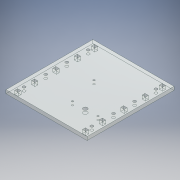
# Autodesk Inventor part: Plano 2
Saved by Autodesk Inventor 2018 (Build 220112000, 112)
## iProperties
Created: 2017-08-31
Part Number: Plano 2
Material: Vidrio
Document SubType Name: Modeling
Designer: Alumno
Density: 2.18 g/cm^3
Appearance: Claro
Author: Alumno
Autodesk Inventor part; units mm, degrees
ref_plane "YZ Plane" through (0, 0, 0) normal (1, 0, 0) x (0, 1, 0)
ref_plane "XZ Plane" through (0, 0, 0) normal (0, 1, 0) x (-1, 0, 0)
ref_plane "XY Plane" through (0, 0, 0) normal (0, 0, 1) x (1, 0, 0)
sketch "Boceto1" plane through (0, 0, 0) normal (0, 0, 1) x (1, 0, 0)
  line L0 (70, -75) -> (-70, -75)
  line L1 (-70, -75) -> (-70, 75)
  line L2 (-70, 75) -> (70, 75)
  line L3 (70, 75) -> (70, -75)
  line L4 (70, -75) -> (-70, 75) construction
  line L5 (-70, -75) -> (70, 75) construction
  point P0 (0, 0)
  dimension "d0" = 140
  dimension "d1" = 150
  constraints: 12 end point, 2 midpoint, 2 parallel, 1 horizontal, 1 perpendicular
  measures "d0" distance of L1.end L2.end
  measures "d1" distance of L0.end L1.end
extrude "Extrusión1" add sketch "Boceto1" along normal blind 6
sketch "Boceto2" plane through (0, 0, 6) normal (0, 0, 1) x (1, 0, 0)
  line L0 (-70, -75) -> (70, -75) projected
  line L1 (70, -75) -> (70, 75) projected
  line L2 (70, 75) -> (-70, 75) projected
  line L3 (-70, 75) -> (-70, -75) projected
  line L4 (70, 75) -> (70, 68.9297)
  line L5 (70, 63.9297) -> (70, 57)
  line L6 (70, 53.65) -> (70, 39.3833)
  line L7 (70, 34.3833) -> (70, 20.1167)
  line L8 (70, 16.7667) -> (70, 2.5)
  line L9 (70, -2.5) -> (70, -16.7667)
  line L10 (70, -20.1167) -> (70, -34.3833)
  line L11 (70, 75) -> (70, 68.9297)
  line L12 (61.5, 68.9297) -> (61.5, 63.9297)
  line L13 (70, 63.9297) -> (70, 57)
  line L14 (70, 53.65) -> (70, 39.3833)
  line L15 (70, 34.3833) -> (70, 20.1167)
  line L16 (70, 16.7667) -> (70, 2.5)
  line L17 (61.5, 2.5) -> (61.5, -2.5)
  line L18 (70, -2.5) -> (70, -16.7667)
  line L19 (70, -20.1167) -> (70, -34.3833)
  line L20 (61.5, -34.3833) -> (61.5, -39.3833)
  line L21 (61.5, -63.5) -> (61.5, -68.5)
  line L22 (61.5, 68.9297) -> (55.5, 68.9297)
  line L23 (55.5, 68.9297) -> (55.5, 63.9297)
  line L24 (55.5, 63.9297) -> (61.5, 63.9297)
  line L25 (61.5, 63.9297) -> (61.5, 68.9297)
  line L26 (61.5, 34.3833) -> (55.5, 34.3833)
  line L27 (55.5, 34.3833) -> (55.5, 39.3833)
  line L28 (55.5, 39.3833) -> (61.5, 39.3833)
  line L29 (61.5, 39.3833) -> (61.5, 34.3833)
  line L30 (55.5, 2.5) -> (61.5, 2.5)
  line L31 (61.5, 2.5) -> (61.5, -2.5)
  line L32 (61.5, -2.5) -> (55.5, -2.5)
  line L33 (55.5, -2.5) -> (55.5, 2.5)
  line L34 (55.5, -34.3833) -> (61.5, -34.3833)
  line L35 (61.5, -34.3833) -> (61.5, -39.3833)
  line L36 (61.5, -39.3833) -> (55.5, -39.3833)
  line L37 (55.5, -39.3833) -> (55.5, -34.3833)
  line L38 (55.5, -68.5) -> (61.5, -68.5)
  line L39 (61.5, -68.5) -> (61.5, -63.5)
  line L40 (61.5, -63.5) -> (55.5, -63.5)
  line L41 (55.5, -63.5) -> (55.5, -68.5)
  dimension "d7" = 5
  dimension "d8" = 6
  dimension "d9" = 5
  dimension "d12" = 6
  dimension "d16" = 6
  dimension "d35" = 8.5
  dimension "d36" = 6
  dimension "d37" = 8.5
  dimension "d40" = 8.5
  dimension "d45" = 8.5
  dimension "d46" = 8.5
  dimension "d47" = 6
  dimension "d48" = 5
  dimension "d49" = 5
  dimension "d50" = 5
  constraints: 76 end point, 10 parallel, 5 horizontal, 5 perpendicular, 2 coincident
  measures "d7" distance of L23.end L22.end
  measures "d8" distance of L27.end L28.end
  measures "d9" distance of L26.end L27.end
  measures "d12" distance of L17.end L32.end
  measures "d16" distance of L20.end L36.end
  measures "d35" distance between parallel lines of L1 L12
  measures "d36" distance of L12.start L22.end
  measures "d37" distance between parallel lines of L1 L29
  measures "d40" distance between parallel lines of L1 L17
  measures "d45" distance between parallel lines of L20 L1
  measures "d46" distance between parallel lines of L1 L21
  measures "d47" distance of L21.start L40.end
  measures "d48" distance of L40.end L38.start
  measures "d49" distance of L20.start L20.end
  measures "d50" distance of L32.end L30.start
extrude "Extrusión2" cut sketch "Boceto2" against normal blind 6 contours L12 L24 L23 L22 | L17 L32 L33 L30 | L20 L36 L37 L34 | L21 L38 L41 L40 | L26 L27 L28 L29
mirror "Simetría1" about plane through (0, 0, 0) normal (1, 0, 0) of "Extrusión2"
sketch "Boceto4" plane through (0, 0, 6) normal (0, 0, 1) x (1, 0, 0)
  line L0 (70, 75) -> (70, 68.9297)
  line L1 (70, 68.9297) -> (65, 68.9297)
  line L2 (65, 68.9297) -> (65, 63.9297)
  line L3 (65, 63.9297) -> (70, 63.9297)
  line L4 (70, 63.9297) -> (70, 57)
  line L5 (70, 53.65) -> (70, 39.3833)
  line L6 (70, 39.3833) -> (65, 39.3833)
  line L7 (65, 39.3833) -> (65, 34.3833)
  line L8 (65, 34.3833) -> (70, 34.3833)
  line L9 (70, 34.3833) -> (70, 20.1167)
  line L10 (70, 16.7667) -> (70, 2.5)
  line L11 (70, 2.5) -> (65, 2.5)
  line L12 (65, 2.5) -> (65, -2.5)
  line L13 (65, -2.5) -> (70, -2.5)
  line L14 (70, -2.5) -> (70, -16.7667)
  line L15 (70, -20.1167) -> (70, -34.3833)
  line L16 (70, -34.3833) -> (65, -34.3833)
  line L17 (65, -34.3833) -> (65, -39.3833)
  line L18 (65, -39.3833) -> (70, -39.3833)
  line L19 (70, -39.3833) -> (70, -53.65)
  line L20 (70, -57) -> (70, -63.5)
  line L21 (70, 75) -> (70, 68.9297)
  line L22 (70, 68.9297) -> (65, 68.9297)
  line L23 (65, 68.9297) -> (65, 63.9297)
  line L24 (65, 63.9297) -> (70, 63.9297)
  line L25 (70, 63.9297) -> (70, 57)
  line L26 (70, 57) -> (76.2, 57)
  line L27 (76.2, 57) -> (76.2, 58.3)
  line L28 (76.2, 58.3) -> (79, 58.3)
  line L29 (79, 58.3) -> (79, 57)
  line L30 (79, 57) -> (82, 57)
  line L31 (82, 57) -> (82, 53.65)
  line L32 (82, 53.65) -> (79, 53.65)
  line L33 (79, 53.65) -> (79, 52.35)
  line L34 (79, 52.35) -> (76.2, 52.35)
  line L35 (76.2, 52.35) -> (76.2, 53.65)
  line L36 (76.2, 53.65) -> (70, 53.65)
  line L37 (70, 53.65) -> (70, 39.3833)
  line L38 (70, 39.3833) -> (65, 39.3833)
  line L39 (65, 39.3833) -> (65, 34.3833)
  line L40 (65, 34.3833) -> (70, 34.3833)
  line L41 (70, 34.3833) -> (70, 20.1167)
  line L42 (70, 20.1167) -> (76.2, 20.1167)
  line L43 (76.2, 20.1167) -> (76.2, 21.4167)
  line L44 (76.2, 21.4167) -> (79, 21.4167)
  line L45 (79, 21.4167) -> (79, 20.1167)
  line L46 (79, 20.1167) -> (82, 20.1167)
  line L47 (82, 20.1167) -> (82, 16.7667)
  line L48 (82, 16.7667) -> (79, 16.7667)
  line L49 (79, 16.7667) -> (79, 15.4667)
  line L50 (79, 15.4667) -> (76.2, 15.4667)
  line L51 (76.2, 15.4667) -> (76.2, 16.7667)
  line L52 (76.2, 16.7667) -> (70, 16.7667)
  line L53 (70, 16.7667) -> (70, 2.5)
  line L54 (70, 2.5) -> (65, 2.5)
  line L55 (65, 2.5) -> (65, -2.5)
  line L56 (65, -2.5) -> (70, -2.5)
  line L57 (70, -2.5) -> (70, -16.7667)
  line L58 (70, -16.7667) -> (76.2, -16.7667)
  line L59 (76.2, -16.7667) -> (76.2, -15.4667)
  line L60 (76.2, -15.4667) -> (79, -15.4667)
  line L61 (79, -15.4667) -> (79, -16.7667)
  line L62 (79, -16.7667) -> (82, -16.7667)
  line L63 (82, -16.7667) -> (82, -20.1167)
  line L64 (82, -20.1167) -> (79, -20.1167)
  line L65 (79, -20.1167) -> (79, -21.4167)
  line L66 (79, -21.4167) -> (76.2, -21.4167)
  line L67 (76.2, -21.4167) -> (76.2, -20.1167)
  line L68 (76.2, -20.1167) -> (70, -20.1167)
  line L69 (70, -20.1167) -> (70, -34.3833)
  line L70 (70, -34.3833) -> (65, -34.3833)
  line L71 (65, -34.3833) -> (65, -39.3833)
  line L72 (65, -39.3833) -> (70, -39.3833)
  line L73 (70, -39.3833) -> (70, -53.65)
  line L74 (70, -53.65) -> (76.2, -53.65)
  line L75 (76.2, -53.65) -> (76.2, -52.35)
  line L76 (76.2, -52.35) -> (79, -52.35)
  line L77 (79, -52.35) -> (79, -53.65)
  line L78 (79, -53.65) -> (82, -53.65)
  line L79 (82, -53.65) -> (82, -57)
  line L80 (82, -57) -> (79, -57)
  line L81 (79, -57) -> (79, -58.3)
  line L82 (79, -58.3) -> (76.2, -58.3)
  line L83 (76.2, -58.3) -> (76.2, -57)
  line L84 (76.2, -57) -> (70, -57)
  line L85 (70, -57) -> (70, -63.5)
  line L86 (70, -63.5) -> (65, -63.5)
  line L87 (65, -63.5) -> (65, -68.5)
  line L88 (65, -68.5) -> (70, -68.5)
  line L89 (70, -68.5) -> (70, -75)
  line L90 (70, 75) -> (70, -75) projected
  line L91 (-61.5, -63.5) -> (-55.5, -63.5) projected
  line L92 (-55.5, -63.5) -> (-55.5, -68.5) projected
  line L93 (-55.5, -68.5) -> (-61.5, -68.5) projected
  line L94 (-61.5, -68.5) -> (-61.5, -63.5) projected
  line L95 (-61.5, 2.5) -> (-55.5, 2.5) projected
  line L96 (-55.5, 2.5) -> (-55.5, -2.5) projected
  line L97 (-55.5, -2.5) -> (-61.5, -2.5) projected
  line L98 (-61.5, -2.5) -> (-61.5, 2.5) projected
  line L99 (-61.5, 34.3833) -> (-61.5, 39.3833) projected
  line L100 (-61.5, 39.3833) -> (-55.5, 39.3833) projected
  line L101 (-55.5, 39.3833) -> (-55.5, 34.3833) projected
  line L102 (-55.5, 34.3833) -> (-61.5, 34.3833) projected
  line L103 (-61.5, -34.3833) -> (-55.5, -34.3833) projected
  line L104 (-55.5, -34.3833) -> (-55.5, -39.3833) projected
  line L105 (-55.5, -39.3833) -> (-61.5, -39.3833) projected
  line L106 (-61.5, -39.3833) -> (-61.5, -34.3833) projected
  line L107 (-55.5, 68.9297) -> (-55.5, 63.9297) projected
  line L108 (-55.5, 63.9297) -> (-61.5, 63.9297) projected
  line L109 (-61.5, 63.9297) -> (-61.5, 68.9297) projected
  line L110 (-61.5, 68.9297) -> (-55.5, 68.9297) projected
  line L111 (55.5, -63.5) -> (61.5, -63.5) projected
  line L112 (61.5, -63.5) -> (61.5, -68.5) projected
  line L113 (61.5, -68.5) -> (55.5, -68.5) projected
  line L114 (55.5, -68.5) -> (55.5, -63.5) projected
  line L115 (55.5, 2.5) -> (61.5, 2.5) projected
  line L116 (61.5, 2.5) -> (61.5, -2.5) projected
  line L117 (61.5, -2.5) -> (55.5, -2.5) projected
  line L118 (55.5, -2.5) -> (55.5, 2.5) projected
  line L119 (61.5, 39.3833) -> (61.5, 34.3833) projected
  line L120 (61.5, 34.3833) -> (55.5, 34.3833) projected
  line L121 (55.5, 34.3833) -> (55.5, 39.3833) projected
  line L122 (55.5, 39.3833) -> (61.5, 39.3833) projected
  line L123 (55.5, -34.3833) -> (61.5, -34.3833) projected
  line L124 (61.5, -34.3833) -> (61.5, -39.3833) projected
  line L125 (61.5, -39.3833) -> (55.5, -39.3833) projected
  line L126 (55.5, -39.3833) -> (55.5, -34.3833) projected
  line L127 (55.5, 63.9297) -> (55.5, 68.9297) projected
  line L128 (55.5, 68.9297) -> (61.5, 68.9297) projected
  line L129 (61.5, 68.9297) -> (61.5, 63.9297) projected
  line L130 (61.5, 63.9297) -> (55.5, 63.9297) projected
  line L131 (-70, -75) -> (70, -75) projected
  line L132 (70, -75) -> (70, 75) projected
  line L133 (70, 75) -> (-70, 75) projected
  line L134 (-70, 75) -> (-70, -75) projected
  circle A0 centre (58.5, 55.325) radius 2.5
  circle A1 centre (58.5, 18.4417) radius 2.5
  circle A2 centre (58.5, -17.8117) radius 2.5
  circle A3 centre (58.5, -55.325) radius 2.5
  line L135 (55.5, -63.5) -> (61.5, -63.5) projected
  point P0 (58.5, -63.5)
  point P1 (58.5, -63.5)
  point P2 (58.5, -63.5)
  point P3 (58.5, 2.5)
  point P4 (58.5, 39.3833)
  dimension "d28" = 5
  dimension "d29" = 5
  dimension "d30" = 5
  dimension "d31" = 5
  constraints: 180 end point, 5 midpoint, 5 vertical alignment, 4 centre point, 1 coincident
  measures "d28" diameter of A0
  measures "d29" diameter of A1
  measures "d30" diameter of A2
  measures "d31" diameter of A3
extrude "Extrusión4" cut sketch "Boceto4" against normal blind 6 contours A0 | A1 | A2 | A3
mirror "Simetría3" about plane through (0, 0, 0) normal (1, 0, 0) of "Extrusión4"
sketch "Boceto5" plane through (0, 0, 6) normal (0, 0, 1) x (1, 0, 0)
  circle A0 centre (-8.2, 15) radius 1.6
  line L0 (70, 75) -> (-70, 75) projected
  line L1 (-70, 75) -> (-70, -75) projected
  line L2 (-70, -75) -> (-70, 75) projected
  circle A1 centre (26.8, -35) radius 3.6
  point P0 (0, 0)
  dimension "d51" = 60
  dimension "d52" = 3.2
  dimension "d53" = 61.8
  dimension "d63" = 7.2
  dimension "d64" = 35
  dimension "d65" = 50
  constraints: 2 centre point
  measures "d51" distance from line of A0.centre L0
  measures "d52" diameter of A0
  measures "d53" distance from line of L1 A0.centre
  measures "d63" diameter of A1
  measures "d64" horizontal distance of A1.centre A0.centre
  measures "d65" vertical distance of A1.centre A0.centre
extrude "Extrusión5" cut sketch "Boceto5" against normal blind 6 contours A0
extrude "Extrusión7" cut sketch "Boceto5" against normal blind 6 contours A1
sketch "Boceto6" plane through (0, 0, 6) normal (0, 0, 1) x (1, 0, 0)
  circle A0 centre (26.8, -35) radius 3.6 projected
  line L0 (4.8, -35) -> (48.8, -35)
  circle A1 centre (4.8, -35) radius 1.5
  circle A2 centre (48.8, -35) radius 1.5
  point P0 (0, 0)
  dimension "d68" = 44
  dimension "d69" = 3
  dimension "d70" = 3
  constraints: 3 coincident, 2 centre point, 2 end point, 1 horizontal, 1 midpoint
  measures "d68" distance of L0.start L0.end
  measures "d69" diameter of A1
  measures "d70" diameter of A2
extrude "Extrusión8" cut sketch "Boceto6" against normal blind 6 contours A1 | A2
